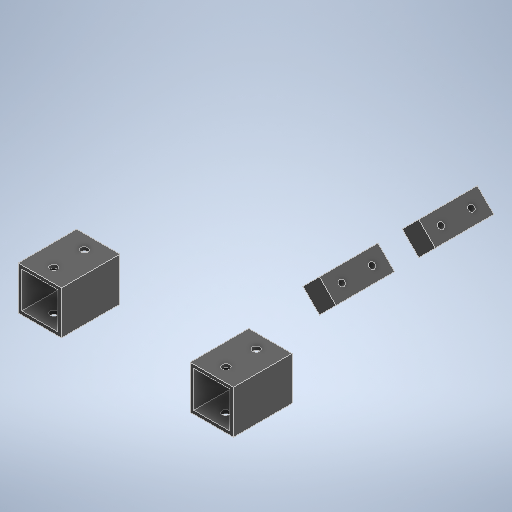
# Autodesk Inventor part: 45_deg
Saved by Autodesk Inventor 2026.1 (Build 301233020, 233B)
## iProperties
Created: 2026-02-01
Part Number: 45_deg
Material: 一般
Document SubType Name: Modeling
Designer: hibik
Density: 1 g/cm^3
Appearance: 既定
Author: hibik
Autodesk Inventor part; units mm, degrees
ref_plane "作業平面1" through (36.75, 0, 0) normal (1, 0, 0) x (0, 1, 0)
sketch "スケッチ1" plane through (0, 0, 0) normal (0, 0, 1) x (1, 0, 0)
  line L0 (36.75, 12.95) -> (36.75, -12.95) projected
  line L1 (29, -7.75) -> (44.5, -7.75)
  line L2 (44.5, -7.75) -> (44.5, 7.75)
  line L3 (44.5, 7.75) -> (29, 7.75)
  line L4 (29, 7.75) -> (29, -7.75)
  line L5 (29, -7.75) -> (44.5, 7.75) construction
  line L6 (44.5, -7.75) -> (29, 7.75) construction
  line L7 (46, -9.25) -> (27.5, -9.25)
  line L8 (27.5, -9.25) -> (27.5, 9.25)
  line L9 (27.5, 9.25) -> (46, 9.25)
  line L10 (46, 9.25) -> (46, -9.25)
  line L11 (46, -9.25) -> (27.5, 9.25) construction
  line L12 (27.5, -9.25) -> (46, 9.25) construction
  point P0 (0, 0)
  point P1 (36.75, 0)
  dimension "d1" = 15.5
  dimension "d2" = 1.5
  constraints: 24 end point, 5 midpoint, 4 parallel, 3 perpendicular, 2 horizontal, 1 horizontal alignment, 1 point on line
  measures "d1" distance of L2.end L3.end
  measures "d2" distance between parallel lines of L9 L3
extrude "押し出し1" add sketch "スケッチ1" along normal blind 25 contours L9 L10 L7 L0 L1 L2 L3 | L0 L3 L4 L1 L7 L8 L9
sketch "スケッチ2" plane through (27.5, 9.25, 0) normal (0, 1, 0) x (1, 0, 0)
  circle A0 centre (9.25, -19) radius 1.6
  line L0 (18.5, -25) -> (0, -25) projected
  circle A1 centre (9.25, -6) radius 1.6
  point P0 (-27.5, 0)
  point P1 (9.25, -25)
  dimension "d5" = 3.2
  dimension "d6" = 6
  dimension "d7" = 3.2
  dimension "d8" = 13
  constraints: 2 centre point, 2 vertical alignment, 1 midpoint
  measures "d5" diameter of A0
  measures "d6" distance from line of L0 A0.centre
  measures "d7" diameter of A1
  measures "d8" distance of A1.centre A0.centre
extrude "押し出し2" cut sketch "スケッチ2" against normal through all
ref_plane "作業平面2" through (27.5, 0, 0) normal (0, 1, 0) x (1, 0, 0)
mirror "ミラー1" about plane through (0, 0, 0) normal (1, 0, 0)
ref_plane "作業平面3" through (-27.5, -40, -9.25) normal (1, 0, 0) x (0, 0, -1)
ref_plane "作業平面4" through (-27.5, 1.5, 40) normal (0, 1, 0) x (1, 0, 0)
ref_plane "作業平面5" through (27.5, -14.25, 0) normal (0, -1, 0) x (1, 0, 0)
ref_plane "作業平面6" through (0, -14.25, 0) normal (0.7071068, -0.7071068, 0) x (0, 0, -1)
sketch "スケッチ10" plane through (0, -14.25, 0) normal (0.7071068, -0.7071068, 0) x (0, 0, -1)
  line L0 (40, 25.0763) -> (65, 25.0763)
  line L1 (65, 25.0763) -> (65, 15.0763)
  line L2 (65, 15.0763) -> (40, 15.0763)
  line L3 (40, 15.0763) -> (40, 25.0763)
  point P0 (0, 10.0763)
  point P1 (40, 20.0763)
  dimension "d78" = 25
  dimension "d79" = 10
  dimension "d81" = 40
  dimension "d90" = 10
  constraints: 8 end point, 2 parallel, 1 horizontal, 1 midpoint, 1 perpendicular
  measures "d78" distance of L1.end L2.end
  measures "d79" distance of L0.end L1.end
  measures "d81" distance from line of point (0, 10.076) L3
  measures "d90" vertical distance of point (0, 10.076) point (40, 20.076)
extrude "押し出し10" add sketch "スケッチ10" along normal blind 10
sketch "スケッチ11" plane through (17.7316, 3.4816, -65) normal (0.7071068, 0.7071068, 0) x (-0.7071068, 0.7071068, 0)
  circle A0 centre (-5, 19) radius 1.3
  circle A1 centre (-5, 6) radius 1.3
  line L0 (0, 25) -> (-10, 25) projected
  line L1 (0, 0) -> (-10, 0) projected
  point P0 (10.0763, 65)
  point P1 (-5, 25)
  point P2 (-5, 25)
  dimension "d84" = 6
  dimension "d85" = 6
  dimension "d86" = 2.6
  constraints: 2 centre point, 2 midpoint, 2 vertical alignment, 1 equal radius
  measures "d84" distance from line of L0 A0.centre
  measures "d85" distance from line of L1 A1.centre
  measures "d86" diameter of A0
extrude "押し出し11" cut sketch "スケッチ11" against normal through all
ref_plane "作業平面8" through (53.0869, 38.8369, -65) normal (0.7071068, 0.7071068, 0) x (-0.7071068, 0.7071068, 0)
sketch "スケッチ13" plane through (53.0869, 38.8369, -65) normal (0.7071068, 0.7071068, 0) x (-0.7071068, 0.7071068, 0)
  circle A0 centre (-5, 19) radius 1.3 projected
  circle A1 centre (-5, 6) radius 1.3 projected
  line L0 (0, 0) -> (0, 25) projected
  line L1 (0, 25) -> (-10, 25) projected
  line L2 (-10, 0) -> (-10, 25) projected
  line L3 (0, 0) -> (-10, 0) projected
  point P0 (10.0763, 65)
extrude "押し出し13" add sketch "スケッチ13" along normal blind 10
equation "\"d5\" = d7"
